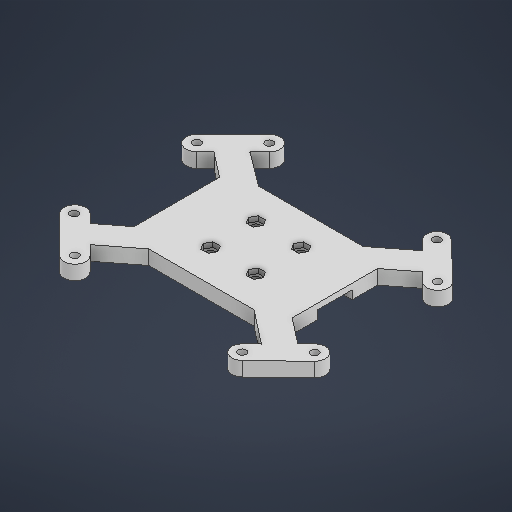
# Autodesk Inventor part: Drone_cross
Saved by Autodesk Inventor 2026.1 (Build 301233000, 233)
## iProperties
Created: 2025-07-26
Part Number: Drone_cross
Material: Generic
Document SubType Name: Modeling
Designer: rohit
Density: 1 g/cm^3
Appearance: Default
Author: rohit
Autodesk Inventor part; units mm, degrees
ref_plane "YZ Plane" through (0, 0, 0) normal (1, 0, 0) x (0, 1, 0)
ref_plane "XZ Plane" through (0, 0, 0) normal (0, 1, 0) x (-1, 0, 0)
ref_plane "Work Plane1" through (0, 1.6, 0) normal (0, 1, 0) x (1, 0, 0)
sketch "Sketch2" plane through (0, 1.6, 0) normal (0, 1, 0) x (1, 0, 0)
  circle A0 centre (23, 7) radius 1.75 projected
  line L0 (21.25, 7) -> (23, 7)
  circle A1 centre (6.8172, 22.8502) radius 1.75 projected
  line L1 (5.0672, 22.8502) -> (6.8172, 22.8502)
  circle A2 centre (6.8172, 77.1499) radius 1.75 projected
  line L2 (5.0672, 77.1499) -> (6.8172, 77.1499)
  circle A3 centre (23, 93) radius 1.75 projected
  line L3 (21.25, 93) -> (23, 93)
  circle A4 centre (97, 7) radius 1.75 projected
  line L4 (95.25, 7) -> (97, 7)
  circle A5 centre (113.1829, 22.8502) radius 1.75 projected
  line L5 (111.4329, 22.8502) -> (113.1829, 22.8502)
  circle A6 centre (113.1829, 77.1499) radius 1.75 projected
  line L6 (111.4329, 77.1499) -> (113.1829, 77.1499)
  circle A7 centre (97, 93) radius 1.75 projected
  line L7 (95.25, 93) -> (97, 93)
  circle A8 centre (23, 7) radius 1.75
  circle A9 centre (6.8172, 22.8502) radius 1.75
  circle A10 centre (6.8172, 77.1499) radius 1.75
  circle A11 centre (23, 93) radius 1.75
  circle A12 centre (97, 93) radius 1.75
  circle A13 centre (113.1829, 77.1499) radius 1.75
  circle A14 centre (113.1829, 22.8502) radius 1.75
  circle A15 centre (97, 7) radius 1.75
  line L8 (6.8172, 22.8502) -> (2.2899, 22.8502)
  line L9 (6.8172, 22.8502) -> (3.6159, 19.6489)
  line L10 (23, 7) -> (18.2375, 7)
  line L11 (23, 7) -> (19.6324, 3.6324)
  line L12 (19.6324, 3.6324) -> (3.6159, 19.6489)
  line L13 (6.8172, 22.8502) -> (10.3511, 26.3841)
  line L14 (23, 7) -> (26.3676, 10.3676)
  line L15 (120, 100.0001) -> (0, 100.0001) projected
  line L16 (113.1829, 77.1499) -> (108.4204, 77.1499)
  line L17 (113.1829, 77.1499) -> (109.8153, 73.7823)
  line L18 (113.1829, 77.1499) -> (116.5505, 80.5175)
  line L19 (97, 93) -> (92.4727, 93)
  line L20 (97, 93) -> (93.7987, 89.7988)
  line L21 (97, 93) -> (100.2013, 96.2013)
  line L22 (116.5505, 80.5175) -> (100.2013, 96.2013)
  line L23 (23, 7) -> (6.8172, 22.8502)
  line L24 (23, 7) -> (23, -11.3324)
  line L25 (23, 7) -> (14.9089, 14.9248)
  line L26 (113.1829, 77.1499) -> (97, 93)
  line L27 (97, 93) -> (97, 106.2617)
  line L28 (97, 93) -> (105.0911, 85.0752)
  line L29 (0, 0) -> (0, 50)
  line L30 (0, 100.0001) -> (0, 0) projected
  line L31 (120, 0) -> (120, 100.0001) projected
  line L32 (19.6324, 96.3676) -> (3.6159, 80.3511)
  line L33 (116.5505, 19.4826) -> (100.2013, 3.7987)
  arc A16 (19.6324, 3.6324) -> (26.3676, 10.3676) centre (23, 7) ccw
  arc A17 (10.3511, 26.3841) -> (3.6159, 19.6489) centre (6.9835, 23.0165) ccw
  line L34 (22.0621, 85.327) -> (37.0786, 74.1625)
  line L35 (83.2604, 74.1625) -> (97.9859, 85.6116)
  arc A18 (3.6159, 80.3511) -> (10.3511, 73.6159) centre (6.9835, 76.9835) ccw
  arc A19 (26.3676, 89.6324) -> (19.6324, 96.3676) centre (23, 93) ccw
  arc A20 (116.5505, 19.4826) -> (109.8153, 26.2178) centre (113.1829, 22.8502) ccw
  line L36 (93.7987, 10.2013) -> (98.0654, 14.3802)
  line L37 (106.0172, 22.4978) -> (109.8153, 26.2178)
  arc A21 (109.8153, 73.7823) -> (116.5505, 80.5175) centre (113.1829, 77.1499) ccw
  arc A22 (100.2013, 96.2013) -> (93.7987, 89.7988) centre (97, 93) ccw
  line L38 (10.3511, 73.6159) -> (14.1298, 77.3946)
  line L39 (22.0621, 85.327) -> (26.3676, 89.6324)
  arc A23 (93.7987, 10.2013) -> (100.2013, 3.7987) centre (97, 7) ccw
  line L40 (15.5072, 21.228) -> (10.3511, 26.3841)
  line L41 (26.3676, 10.3676) -> (22.2406, 14.4946)
  line L42 (109.8153, 73.7823) -> (106.0611, 77.5364)
  line L43 (97.9859, 85.6116) -> (93.7987, 89.7988)
  line L44 (22.2406, 14.4946) -> (15.5072, 21.228)
  line L45 (6.8172, 22.8502) -> (6.8172, 36.0698)
  line L46 (31.9559, 119.5066) -> (31.9559, 155.0666)
  line L47 (31.9559, 155.0666) -> (-39.1641, 155.0666)
  line L48 (-39.1641, 155.0666) -> (-39.1641, 119.5066)
  line L49 (-39.1641, 119.5066) -> (31.9559, 119.5066)
  line L50 (24.3041, 175.988) -> (54.7841, 175.988)
  line L51 (54.7841, 175.988) -> (54.7841, 203.928)
  line L52 (54.7841, 203.928) -> (24.3041, 203.928)
  line L53 (24.3041, 203.928) -> (24.3041, 175.988)
  line L54 (83.3672, 25.8376) -> (36.8534, 25.8376)
  line L55 (83.2604, 74.1625) -> (37.0786, 74.1625)
  line L56 (94.925, 31.1303) -> (94.925, 68.8698)
  line L57 (22.2406, 14.4946) -> (36.8534, 25.8376)
  line L58 (98.0654, 14.3802) -> (83.3672, 25.8376)
  line L59 (0, 50) -> (34.6, 50)
  line L60 (103.7116, 86.4264) -> (120, 100.0001)
  line L61 (106.0611, 77.5364) -> (94.925, 68.8698)
  line L62 (34.6, 50) -> (109.6103, 50)
  line L63 (14.1298, 77.3946) -> (25.075, 68.8698)
  line L64 (106.0611, 22.4637) -> (94.925, 31.1303)
  line L65 (14.1298, 22.6054) -> (25.075, 31.1303)
  line L66 (25.075, 68.8698) -> (25.075, 31.1303)
  dimension "d20" = 45
  dimension "d21" = 45
  dimension "d22" = 45
  dimension "d23" = 45
  dimension "d26" = 50
  dimension "d41" = 16.0165
  dimension "d42" = 4.7625
  dimension "d43" = 4.7625
  dimension "d44" = 6.7335
  dimension "d45" = 134.405
  dimension "d49" = 71.12
  dimension "d50" = 35.56
  dimension "d53" = 27.94
  dimension "d54" = 30.48
  constraints: 128 end point, 16 centre point, 16 point on circle, 13 horizontal, 12 coincident, 10 point on line, 8 horizontal alignment, 5 perpendicular, 5 tangent, 4 parallel, 4 symmetric about line, 2 collinear, 1 vertical, 16 other
  measures "d20" angle of L9 L8
  measures "d21" angle of L10 L11
  measures "d22" angle of L17 L16
  measures "d23" angle of L20 L19
  measures "d26" distance of L29.start L29.end
  measures "d41" horizontal distance of L11.end L9.end
  measures "d42" radius of A17
  measures "d43" radius of A16
  measures "d44" horizontal distance of L41.end L40.start
  measures "d45" angle of L45 L23
  measures "d49" distance of L48.end L46.start
  measures "d50" distance of L47.end L48.end
  measures "d53" distance of L52.end L50.start
  measures "d54" distance of L51.end L52.end
extrude "Extrusion4" add sketch "Sketch2" along normal blind 6.35 contours A0 L14 A16 L24 | A0 L23 A1 L13 L40 L44 L41 L14 | L24 A16 L11 A0 | A0 L11 L12 L9 A1 L23 | L44 L40 L65 L66 L59 L62 L56 L64 L37 A20 L33 A23 L36 L58 L54 L57 | A17 L45 A1 L9 | A17 L13 A1 L45 | L66 L63 L38 A18 L32 A19 L39 L34 L55 L35 L43 L20 A7 L26 A6 L17 L42 L61 L56 L62 L59 | A22 L21 A7 L27 | L27 A7 L19 A22 | L60 L26 A7 L21 L22 | L22 L18 A6 L26 L60 | L19 A7 L20 A22 | L17 A6 L18 A21
sketch "Sketch18" plane through (0, 1.6, 0) normal (0, -1, 0) x (1, 0, 0)
  line L0 (83.2604, -74.1625) -> (37.0786, -74.1625) projected
  line L1 (22.2406, -14.4946) -> (36.8534, -25.8376) projected
  line L2 (94.925, -74.1625) -> (25.075, -74.1625)
  line L3 (25.075, -74.1625) -> (25.075, -25.8376)
  line L4 (25.075, -25.8376) -> (94.925, -25.8376)
  line L5 (94.925, -25.8376) -> (94.925, -74.1625)
  line L6 (75, -66) -> (45, -66)
  line L7 (45, -66) -> (45, -34.0001)
  line L8 (45, -34.0001) -> (75, -34.0001)
  line L9 (75, -34.0001) -> (75, -66)
  line L10 (70, -60) -> (50, -60)
  line L11 (50, -60) -> (50, -40)
  line L12 (50, -40) -> (70, -40)
  line L13 (70, -40) -> (70, -60)
  line L14 (0, -99.1742) -> (0, 0)
  circle A0 centre (50, -60) radius 1.75
  circle A1 centre (50, -40) radius 1.75
  circle A2 centre (70, -60) radius 1.75
  circle A3 centre (70, -40) radius 1.75
  point P0 (94.925, -71.2652)
  point P1 (25.075, -28.6863)
  dimension "d111" = 29.9999
  dimension "d112" = 48.3249
  dimension "d113" = 69.85
  dimension "d114" = 31.9999
  dimension "d115" = 19.925
  dimension "d118" = 20
  dimension "d119" = 20
  dimension "d120" = 5
  dimension "d121" = 25.075
  dimension "d122" = 6
  dimension "d124" = 3.5
  dimension "d125" = 3.5
  dimension "d126" = 3.5
  dimension "d127" = 3.5
  dimension "d130" = 8.1625
  constraints: 26 end point, 6 parallel, 4 centre point, 4 coincident, 3 horizontal, 3 perpendicular, 1 vertical
  measures "d111" distance of L7.end L8.end
  measures "d112" distance of L2.end L3.end
  measures "d113" distance of L2.start L2.end
  measures "d114" distance of L6.end L7.end
  measures "d115" distance between parallel lines of L5 L9
  measures "d118" distance of L10.start L10.end
  measures "d119" distance of L10.end L11.end
  measures "d120" distance between parallel lines of L9 L13
  measures "d121" distance between parallel lines of L14 L3
  measures "d122" distance between parallel lines of L8 L12
  measures "d124" diameter of A0
  measures "d125" diameter of A1
  measures "d126" diameter of A2
  measures "d127" diameter of A3
  measures "d130" distance between parallel lines of L0 L6
extrude "Extrusion15" cut sketch "Sketch18" against normal blind 12.9499 contours A0 L11 L10 | L10 L11 A0 | A2 L13 L10 | L10 L13 A2 | A1 L12 L11 | L11 L12 A1 | A3 L12 L13 | L13 L12 A3
sketch "Sketch25" plane through (0, 7.95, 0) normal (0, 1, 0) x (1, 0, 0)
  circle A0 centre (70, 40) radius 1.75 projected
  line L0 (70, 40) -> (66.826, 39.9225)
  line L1 (70, 40) -> (68.3459, 42.7101)
  line L2 (70, 40) -> (71.5199, 42.7876)
  line L3 (70, 40) -> (73.1741, 40.0775)
  line L4 (70, 40) -> (71.6542, 37.29)
  line L5 (70, 40) -> (68.4801, 37.2125)
  line L6 (73.1741, 40.0775) -> (71.5199, 42.7876)
  line L7 (71.5199, 42.7876) -> (68.3459, 42.7101)
  line L8 (66.826, 39.9225) -> (68.3459, 42.7101)
  line L9 (68.4801, 37.2125) -> (66.826, 39.9225)
  line L10 (71.6542, 37.29) -> (73.1741, 40.0775)
  line L11 (71.6542, 37.29) -> (68.4801, 37.2125)
  line L12 (70, 60) -> (66.826, 59.9225)
  line L13 (70, 60) -> (68.3459, 62.7101)
  line L14 (70, 60) -> (71.5199, 62.7876)
  line L15 (70, 60) -> (73.1741, 60.0775)
  line L16 (70, 60) -> (71.6542, 57.29)
  line L17 (70, 60) -> (68.4801, 57.2125)
  line L18 (73.1741, 60.0775) -> (71.5199, 62.7876)
  line L19 (71.5199, 62.7876) -> (68.3459, 62.7101)
  line L20 (66.826, 59.9225) -> (68.3459, 62.7101)
  line L21 (68.4801, 57.2125) -> (66.826, 59.9225)
  line L22 (71.6542, 57.29) -> (73.1741, 60.0775)
  line L23 (71.6542, 57.29) -> (68.4801, 57.2125)
  line L24 (50, 60) -> (46.8259, 59.9225)
  line L25 (50, 60) -> (48.3459, 62.7101)
  line L26 (50, 60) -> (51.5199, 62.7876)
  line L27 (50, 60) -> (53.1741, 60.0775)
  line L28 (50, 60) -> (51.6542, 57.29)
  line L29 (50, 60) -> (48.4801, 57.2125)
  line L30 (53.1741, 60.0775) -> (51.5199, 62.7876)
  line L31 (51.5199, 62.7876) -> (48.3459, 62.7101)
  line L32 (46.8259, 59.9225) -> (48.3459, 62.7101)
  line L33 (48.4801, 57.2125) -> (46.8259, 59.9225)
  line L34 (51.6542, 57.29) -> (53.1741, 60.0775)
  line L35 (51.6542, 57.29) -> (48.4801, 57.2125)
  line L36 (50, 40) -> (46.8259, 39.9225)
  line L37 (50, 40) -> (48.3459, 42.7101)
  line L38 (50, 40) -> (51.5199, 42.7876)
  line L39 (50, 40) -> (53.1741, 40.0775)
  line L40 (50, 40) -> (51.6542, 37.29)
  line L41 (50, 40) -> (48.4801, 37.2125)
  line L42 (53.1741, 40.0775) -> (51.5199, 42.7876)
  line L43 (51.5199, 42.7876) -> (48.3459, 42.7101)
  line L44 (46.8259, 39.9225) -> (48.3459, 42.7101)
  line L45 (48.4801, 37.2125) -> (46.8259, 39.9225)
  line L46 (51.6542, 37.29) -> (53.1741, 40.0775)
  line L47 (51.6542, 37.29) -> (48.4801, 37.2125)
  circle A1 centre (70, 60) radius 1.75 projected
  line L48 (70, 60) -> (70, 63.9973)
  circle A2 centre (50, 60) radius 1.75 projected
  line L49 (50, 60) -> (50, 63.553)
  circle A3 centre (50, 40) radius 1.75 projected
  line L50 (50, 40) -> (49.9075, 43.787)
  point P0 (0, 0)
  dimension "d241" = 34.925
  dimension "d244" = 15.2456
  dimension "d245" = 10.16
  dimension "d168" = 3.175
  dimension "d169" = 3.175
  dimension "d170" = 3.175
  dimension "d171" = 3.175
  dimension "d172" = 3.175
  dimension "d173" = 3.175
  dimension "d174" = 60
  dimension "d175" = 60
  dimension "d176" = 60
  dimension "d177" = 60
  dimension "d178" = 60
  dimension "d179" = 3.175
  dimension "d180" = 3.175
  dimension "d181" = 3.175
  dimension "d182" = 3.175
  dimension "d183" = 3.175
  dimension "d184" = 3.175
  dimension "d185" = 60
  dimension "d186" = 60
  dimension "d187" = 60
  dimension "d188" = 60
  dimension "d189" = 60
  dimension "d190" = 3.175
  dimension "d191" = 3.175
  dimension "d192" = 3.175
  dimension "d193" = 3.175
  dimension "d194" = 3.175
  dimension "d195" = 3.175
  dimension "d196" = 60
  dimension "d197" = 60
  dimension "d198" = 60
  dimension "d199" = 60
  dimension "d200" = 60
  dimension "d201" = 3.175
  dimension "d202" = 3.175
  dimension "d203" = 3.175
  dimension "d204" = 3.175
  dimension "d205" = 3.175
  dimension "d206" = 3.175
  dimension "d207" = 60
  dimension "d208" = 60
  dimension "d209" = 60
  dimension "d210" = 60
  dimension "d211" = 60
  constraints: 102 end point, 12 parallel, 8 point on line, 2 vertical
  measures "d168" distance of L0.start L0.end
  measures "d169" distance of L0.start L1.end
  measures "d170" distance of L0.start L2.end
  measures "d171" distance of L0.start L3.end
  measures "d172" distance of L0.start L4.end
  measures "d173" distance of L0.start L5.end
  measures "d174" angle of L1 L0
  measures "d175" angle of L2 L1
  measures "d176" angle of L3 L2
  measures "d177" angle of L4 L3
  measures "d178" angle of L4 L5
  measures "d179" distance of L12.start L12.end
  measures "d180" distance of L12.start L13.end
  measures "d181" distance of L12.start L14.end
  measures "d182" distance of L12.start L15.end
  measures "d183" distance of L12.start L23.start
  measures "d184" distance of L12.start L21.start
  measures "d185" angle of L13 L12
  measures "d186" angle of L14 L13
  measures "d187" angle of L15 L14
  measures "d188" angle of L16 L15
  measures "d189" angle of L16 L17
  measures "d190" distance of L24.start L24.end
  measures "d191" distance of L24.start L25.end
  measures "d192" distance of L24.start L26.end
  measures "d193" distance of L24.start L27.end
  measures "d194" distance of L24.start L35.start
  measures "d195" distance of L24.start L33.start
  measures "d196" angle of L25 L24
  measures "d197" angle of L26 L25
  measures "d198" angle of L27 L26
  measures "d199" angle of L28 L27
  measures "d200" angle of L28 L29
  measures "d201" distance of L36.start L36.end
  measures "d202" distance of L36.start L37.end
  measures "d203" distance of L36.start L38.end
  measures "d204" distance of L36.start L39.end
  measures "d205" distance of L36.start L47.start
  measures "d206" distance of L36.start L45.start
  measures "d207" angle of L37 L36
  measures "d208" angle of L38 L37
  measures "d209" angle of L39 L38
  measures "d210" angle of L40 L39
  measures "d211" angle of L40 L41
extrude "Extrusion22" cut sketch "Sketch25" against normal blind 2.159 contours A0 L3 L10 L4 | A0 L2 L6 L3 | L4 L11 L5 A0 | A0 L1 L7 L2 | L5 L9 L0 A0 | A0 L0 L8 L1 | A1 L17 L21 L12 | L12 L20 L13 A1 | L13 L19 L48 A1 | A1 L48 L19 L14 | L14 L18 L15 A1 | L15 L22 L16 A1 | L16 L23 L17 A1 | A2 L29 L33 L24 | L24 L32 L25 A2 | L25 L31 L49 A2 | A2 L49 L31 L26 | L26 L30 L27 A2 | L27 L34 L28 A2 | L28 L35 L29 A2 | A3 L41 L45 L36 | L36 L44 L37 A3 | L37 L43 L50 A3 | A3 L50 L43 L38 | L38 L42 L39 A3 | L39 L46 L40 A3 | L40 L47 L41 A3
sketch "Sketch30" plane through (0, 1.6, 0) normal (0, -1, 0) x (1, 0, 0)
  line L0 (36.8534, -25.8376) -> (83.3672, -25.8376) projected
  line L1 (36.8534, -25.8376) -> (26.6397, -25.8376)
  line L2 (26.6397, -25.8376) -> (19.1384, -25.8376)
  line L3 (25.075, -28.6863) -> (15.5072, -21.228) projected
  line L4 (25.075, -28.6863) -> (25.075, -19.9564)
  line L5 (25.075, -71.2738) -> (25.075, -28.6863) projected
  line L6 (25.075, -71.2738) -> (25.075, -79.7824)
  line L7 (83.2604, -74.1625) -> (37.0786, -74.1625) projected
  line L8 (37.0786, -74.1625) -> (22.4586, -74.1625)
  line L9 (25.075, -25.8376) -> (35.235, -25.8376)
  line L10 (35.235, -25.8376) -> (35.235, -74.1625)
  line L11 (35.235, -74.1625) -> (25.075, -74.1625)
  line L12 (25.075, -74.1625) -> (25.075, -25.8376)
  line L13 (25.075, -25.8376) -> (25.075, -50.0057)
  line L14 (25.075, -50.0057) -> (35.235, -50)
  line L15 (35.235, -50) -> (35.235, -42.38)
  line L16 (25.075, -50.0057) -> (25.075, -57.6257)
  line L17 (35.235, -42.38) -> (25.075, -42.38)
  line L18 (25.075, -42.38) -> (25.075, -57.6257)
  line L19 (25.075, -57.6257) -> (35.235, -57.6257)
  line L20 (35.235, -57.6257) -> (35.235, -42.38)
  line L21 (83.3672, -25.8376) -> (97.0518, -25.8376)
  line L22 (94.925, -28.7897) -> (94.925, -24.641)
  line L23 (94.925, -25.8376) -> (60, -25.8376)
  line L24 (60, -25.8376) -> (60, -91.5414)
  line L25 (94.925, -25.8376) -> (94.925, -50.0057)
  line L26 (94.925, -50.0057) -> (94.925, -57.6257)
  line L27 (84.765, -42.38) -> (94.925, -42.38)
  line L28 (94.925, -57.6257) -> (84.765, -57.6257)
  line L29 (84.765, -57.6257) -> (84.765, -42.38)
  point P0 (0, 0)
  dimension "d235" = 10.16
  dimension "d236" = 24.1681
  dimension "d237" = 7.62
  dimension "d238" = 7.62
  dimension "d241" = 34.925
  dimension "d244" = 15.2456
  dimension "d245" = 10.16
  constraints: 52 end point, 11 point on line, 5 perpendicular, 5 symmetric about line, 4 parallel, 3 horizontal, 2 vertical, 1 midpoint
  measures "d235" distance of L10.end L11.end
  measures "d236" distance of L9.start L13.end
  measures "d237" distance of L14.end L15.end
  measures "d238" distance of L13.end L16.end
  measures "d241" distance of L23.start L23.end
  measures "d244" distance of L19.end L15.end
  measures "d245" distance of L16.end L19.end
extrude "Extrusion30" cut sketch "Sketch30" against normal blind 3.81 contours L25 L26 L28 L29 L27 | L10 L14 L5 L17 | L10 L19 L5 L14
body "Solid2"
